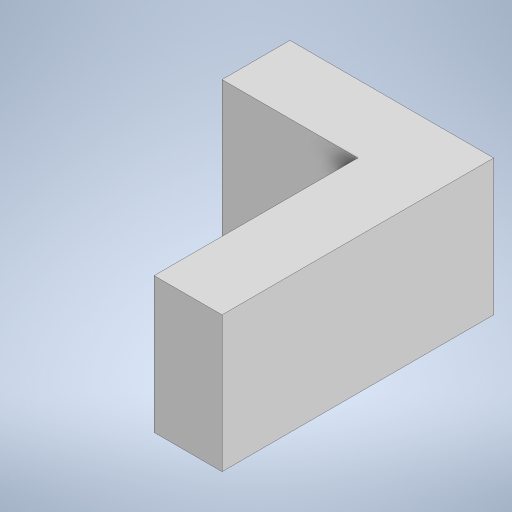
# Autodesk Inventor part: primeiro desenho
Saved by Autodesk Inventor 2024 (Build 280153000, 153)
## iProperties
Created: 2023-09-11
Part Number: primeiro desenho
Material: Generic
Document SubType Name: Sheet Metal
Designer: LORAC
Density: 1 g/cm^3
Sheet Metal Rule: Default_mm
Appearance: Default
Author: LORAC
Autodesk Inventor part; units mm, degrees
ref_plane "YZ Plane" through (0, 0, 0) normal (1, 0, 0) x (0, 1, 0)
ref_plane "XZ Plane" through (0, 0, 0) normal (0, 1, 0) x (-1, 0, 0)
ref_plane "XY Plane" through (0, 0, 0) normal (0, 0, 1) x (1, 0, 0)
sketch "Sketch1" plane through (0, 0, 0) normal (0, 1, 0) x (-1, 0, 0)
  line L0 (0, 0) -> (0, -20)
  line L1 (0, -20) -> (15, -20)
  line L2 (15, -20) -> (15, -15)
  line L3 (15, -15) -> (5, -15)
  line L4 (5, -15) -> (5, 0)
  line L5 (5, 0) -> (0, 0)
  dimension "d0" = 20
  dimension "d2" = 15
  dimension "d4" = 5
  dimension "d5" = 10
  dimension "d6" = 15
  constraints: 12 end point, 3 vertical, 2 horizontal
  measures "d0" distance of L0.start L0.end
  measures "d2" distance of L0.end L1.end
  measures "d4" distance of L1.end L2.end
  measures "d5" distance of L2.end L3.end
  measures "d6" distance of L3.end L4.end
extrude "Extrusion1" add sketch "Sketch1" along normal blind 10
equation "\"BendRadius\" = Thickness"
equation "\"BendReliefWidth\" = Thickness"
equation "\"BendReliefDepth\" = 0.5 * Thickness"
equation "\"CornerReliefSize\" = 4 * Thickness"
equation "\"MinimumRemnant\" = 2 * Thickness"
equation "\"TransitionRadius\" = BendRadius"
equation "\"JacobiRadiusSize\" = BendRadius"
equation "\"GapSize\" = Thickness"
equation "\"Thickness\" = 0.5"
body "Solid1"
